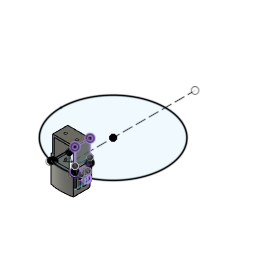
Aquazepp_Relais_Holder v4 (Autodesk Fusion 360 design; units mm, degrees)
Autodesk Fusion 360 part; units mm, degrees
sketch "Skizze1" plane through (0, 0, 0) normal (0, 0, 1) x (1, 0, 0)
  line L0 (-25.6418, 33.3344) -> (-25.6418, 4.3344)
  line L1 (-25.6418, 4.3344) -> (11.3582, 4.3344)
  line L2 (11.3582, 4.3344) -> (11.3582, 33.3344)
  line L3 (-28.6418, 33.3344) -> (-28.6418, 1.3344)
  line L4 (-28.6418, 1.3344) -> (14.3582, 1.3344)
  line L5 (14.3582, 1.3344) -> (14.3582, 33.3344)
  line L6 (-28.6418, 33.3344) -> (-25.6418, 33.3344)
  line L7 (11.3582, 33.3344) -> (14.3582, 33.3344)
  dimension "d1" = 29
  dimension "d2" = 37
  dimension "d3" = 29
  dimension "d4" = 3
  constraint vertical L0
  constraint perpendicular L0 L1
  constraint perpendicular L1 L2
  constraint perpendicular L0 L6
  measures "d1" distance of L0.start L0.end
  measures "d2" distance of L0.end L1.end
  measures "d3" distance of L1.end L2.end
extrude "Extrusion1" add sketch "Skizze1" along normal blind 39 makes body 1
sketch "Skizze2" plane through (14.3582, 0, 0) normal (1, 0, 0) x (0, 1, 0)
  line L0 (1.3344, 0) -> (33.3344, 0)
  line L1 (33.3344, 0) -> (33.3344, 39)
  line L2 (33.3344, 39) -> (1.3344, 39)
  line L3 (1.3344, 39) -> (1.3344, 0)
  line L4 (1.3344, 39) -> (33.3344, 39)
  line L5 (1.3344, 0) -> (1.3344, 39)
  line L6 (1.3344, 0) -> (33.3344, 0)
  line L7 (33.3344, 0) -> (33.3344, 39)
  circle A0 centre (14.3344, 30) radius 2.5
  circle A1 centre (26.3344, 30) radius 2.5
  circle A2 centre (14.3344, 18) radius 2.5
  circle A3 centre (26.3344, 18) radius 2.5
  dimension "d7" = 5
  dimension "d10" = 12
  dimension "d11" = -12
  dimension "d12" = 9
  dimension "d13" = 13
  measures "d7" diameter of A0
  measures "d12" distance of L4 A0.centre
  measures "d13" distance of L5 A0.centre
sketch "Skizze3" plane through (-28.6418, 0, 0) normal (-1, 0, 0) x (0, -1, 0)
  line L0 (-33.3344, 0) -> (-1.3344, 0)
  line L1 (-1.3344, 0) -> (-1.3344, 39)
  line L2 (-1.3344, 39) -> (-33.3344, 39)
  line L3 (-33.3344, 39) -> (-33.3344, 0)
  circle A0 centre (-26.3344, 30) radius 2.5
  circle A1 centre (-14.3344, 18) radius 2.5
extrude "Extrusion2" cut sketch "Skizze2" against normal blind 5 contours A0 | A3 bodies 1
extrude "Extrusion3" cut sketch "Skizze3" against normal blind 5 contours A0 | A1 bodies 1
sketch "Skizze4" plane through (0, 0, 39) normal (0, 0, 1) x (-1, 0, 0)
  line L0 (28.6418, -33.3344) -> (28.6418, -1.3344)
  line L1 (28.6418, -1.3344) -> (-14.3582, -1.3344)
  line L2 (-14.3582, -1.3344) -> (-14.3582, -33.3344)
  line L3 (-14.3582, -33.3344) -> (-11.3582, -33.3344)
  line L4 (-11.3582, -33.3344) -> (-11.3582, -4.3344)
  line L5 (-11.3582, -4.3344) -> (25.6418, -4.3344)
  line L6 (25.6418, -4.3344) -> (25.6418, -33.3344)
  line L7 (25.6418, -33.3344) -> (28.6418, -33.3344)
  circle A0 centre (7.1418, -99.3344) radius 100.5
  line L8 (25.6418, -33.3344) -> (-11.3582, -4.3344) construction
  line L9 (-11.3582, -33.3344) -> (25.6418, -4.3344) construction
  line L10 (7.1418, -18.8344) -> (7.1418, -257.1246) construction
  line L11 (28.6418, -1.3344) -> (28.6418, 1.2)
  line L12 (-14.3582, -1.3344) -> (-14.3582, 1)
  dimension "d18" = 201
  dimension "d19" = 98
  constraint coincident L6.end L7.start
  constraint coincident L4.end L5.start
  constraint coincident L3.end L4.start
  constraint coincident L5.end L6.start
  constraint midpoint L9 L10.start
  constraint perpendicular L5 L10
  constraint coincident A0.centre L10
  constraint coincident L0.end L1.start
  constraint perpendicular L1 L11
  constraint coincident L1.end L2.start
  constraint perpendicular L1 L12
  measures "d18" diameter of A0
  measures "d19" distance of L1 A0.centre
extrude "Extrusion4" add sketch "Skizze4" against normal blind 39 contours L1 A0 L11 L12 bodies 1
ref_plane "Arbeitsebene1" through (-7.1418, 12.8935, 41) normal (0, 0, 1) x (1, 0, 0)
sketch "Skizze5" plane through (-7.1418, 12.8935, 41) normal (0, 0, 1) x (1, 0, 0)
  line L0 (-18.5, 20.4409) -> (-18.5, -8.5591)
  line L1 (18.5, -8.5591) -> (18.5, 20.4409)
  line L2 (-21.5, 20.4409) -> (-21.5, -11.5591)
  line L3 (-21.5, -11.5591) -> (21.5, -11.5591)
  line L4 (-18.5, -8.5591) -> (18.5, -8.5591)
  line L5 (18.5, 20.4409) -> (21.5, 20.4409)
  line L6 (-21.5, 20.4409) -> (-18.5, 20.4409)
  line L7 (21.5, -11.5591) -> (21.5, 20.4409)
  line L8 (-18.5, -8.5591) -> (-21.5, -8.5591)
  line L9 (18.5, -8.5591) -> (21.5, -8.5591)
  constraint coincident L0.end L4.start
  constraint coincident L2 L8.end
  constraint perpendicular L2 L8
  constraint coincident L1.start L4.end
  constraint coincident L7 L9.end
  constraint perpendicular L7 L9
extrude "Extrusion5" add sketch "Skizze5" along normal blind 40 separate body contours L0 L2 L6 L8 | L1 L5 L7 L9 makes body 2 at (-25.6418, 14.001, 67.6667) makes body 3 at (11.3582, 23.6677, 67.6667)
sketch "Skizze6" plane through (0, 0, 81) normal (0, 0, 1) x (-1, 0, 0)
  line L0 (28.6418, -33.3344) -> (28.6418, -4.3344)
  line L1 (-14.3582, -4.3344) -> (-14.3582, -33.3344)
  line L2 (-14.3582, -33.3344) -> (-11.3582, -33.3344)
  line L3 (-11.3582, -33.3344) -> (-11.3582, -4.3344)
  line L4 (25.6418, -4.3344) -> (25.6418, -33.3344)
  line L5 (25.6418, -33.3344) -> (28.6418, -33.3344)
  line L6 (-14.3582, -1.3344) -> (-14.3582, -33.3344)
  line L7 (-11.3582, -4.3344) -> (-11.3582, -33.3344)
  line L8 (-11.3582, -33.3344) -> (-14.3582, -33.3344)
  line L9 (28.6418, -33.3344) -> (25.6418, -33.3344)
  line L10 (28.6418, -33.3344) -> (28.6418, -1.3344)
  line L11 (25.6418, -33.3344) -> (25.6418, -4.3344)
  line L12 (25.6418, -4.3344) -> (-11.3582, -4.3344)
  line L13 (28.6418, -1.3344) -> (-14.3582, -1.3344)
  line L14 (25.6418, -33.3344) -> (-11.3582, -33.3344)
  line L15 (-11.3582, -4.3344) -> (-14.3582, -4.3344)
  line L16 (28.6418, -4.3344) -> (25.6418, -4.3344)
  circle A0 centre (-3.6582, -18.7894) radius 2.5
  line L17 (25.6418, -33.3344) -> (-11.3582, -4.3344) construction
  line L18 (-11.3582, -33.3344) -> (25.6418, -4.3344) construction
  line L19 (7.1418, -18.8344) -> (7.1418, -24) construction
  line L20 (7.1418, -18.8344) -> (0, -18.8344) construction
  circle A1 centre (17.9418, -18.7894) radius 2.5
  dimension "d29" = 5
  dimension "d32" = 5
  dimension "d33" = 21.6
  constraint coincident L4.end L5.start
  constraint coincident L2.end L3.start
  constraint coincident L3.end L7.start
  constraint coincident L4.start L11.end
  constraint midpoint L18 L19.start
  constraint parallel L11 L19
  constraint perpendicular L19 L20
  constraint symmetric A0 L19 A1
  measures "d29" diameter of A0
  measures "d32" diameter of A1
  measures "d33" distance of A0.centre A1.centre
extrude "Extrusion6" add sketch "Skizze6" against normal blind 3 contours L3 L4 L7 L11 L12 L14 bodies 2 3
extrude "Extrusion7" add sketch "Skizze6" 1 faces at (-10.4374, 29.2618, 81) along normal blind 1 contours A0 | A1 on bodies 2 bodies 2
sketch "Skizze7" plane through (14.3582, 0, 0) normal (1, 0, 0) x (0, 1, 0)
  line L0 (4.3344, 41) -> (33.3344, 41)
  line L1 (33.3344, 41) -> (33.3344, 82)
  line L2 (33.3344, 82) -> (4.3344, 82)
  line L3 (4.3344, 82) -> (4.3344, 41)
  line L4 (4.3344, 41) -> (4.3344, 82)
  line L5 (33.3344, 41) -> (33.3344, 82)
  circle A0 centre (14.3344, 30) radius 2.5
  circle A1 centre (26.3344, 18) radius 2.5
  line L6 (4.3344, 41) -> (4.3344, 11)
  line L7 (33.3344, 41) -> (33.3344, 11)
  line L8 (33.3344, 11) -> (4.3344, 11)
  line L9 (11.8344, 30) -> (11.8344, 11)
  circle A2 centre (26.3344, 30) radius 2.5
  circle A3 centre (26.3344, 18) radius 2.5
  line L10 (16.8344, 30.0061) -> (16.8804, 11)
  line L11 (23.8344, 30.0061) -> (23.7883, 11)
  line L12 (28.8344, 30.0061) -> (28.8804, 11)
  line L13 (4.3344, 50.1435) -> (33.3344, 50.1435)
  constraint coincident L0.start L3.end
  constraint perpendicular L0 L6
  constraint coincident L0.end L1.start
  constraint parallel L4 L7
  constraint perpendicular L6 L8
  constraint coincident A0 L9.start
  constraint coincident L8 L9.end
  constraint tangent A0 L9
  constraint perpendicular L8 L9
  constraint coincident A0 L10.start
  constraint coincident L8 L10.end
  constraint tangent A0 L10
  constraint coincident A2 L11.start
  constraint coincident L8 L11.end
  constraint tangent A2 L11
  constraint coincident A2 L12.start
  constraint coincident L8 L12.end
  constraint tangent A2 L12
  constraint coincident L3 L13.start
  constraint coincident L1 L13.end
  constraint perpendicular L1 L13
extrude "Extrusion8" add sketch "Skizze7" along normal blind 3 separate body contours L0 L1 L3 L4 L5 L13 | L0 A0 L6 L7 L8 L9 A2 L10 L11 L12 makes body 4
sketch "Skizze8" plane through (-28.6418, 0, 0) normal (-1, 0, 0) x (0, -1, 0)
  line L0 (-33.3344, 41) -> (-4.3344, 41)
  line L1 (-4.3344, 41) -> (-4.3344, 82)
  line L2 (-4.3344, 82) -> (-33.3344, 82)
  line L3 (-33.3344, 82) -> (-33.3344, 41)
  line L4 (-4.3344, 50.1435) -> (-33.3344, 50.1435)
  line L5 (-33.3344, 41) -> (-33.3344, 82)
  line L6 (-4.3344, 41) -> (-4.3344, 82)
  line L7 (-4.3344, 41) -> (-4.3344, 11)
  line L8 (-33.3344, 41) -> (-33.3344, 11)
  circle A0 centre (-26.3344, 30) radius 2.5
  line L9 (-28.8344, 30.0061) -> (-28.8804, 11)
  line L10 (-23.8344, 30.0061) -> (-23.7883, 11)
  circle A1 centre (-14.3344, 30) radius 2.5
  line L11 (-16.8344, 30.0061) -> (-16.8804, 11)
  line L12 (-11.8344, 30) -> (-11.8344, 11)
  line L13 (-33.3344, 11) -> (-4.3344, 11)
extrude "Extrusion9" add sketch "Skizze8" along normal blind 3 separate body contours L0 L1 L3 L4 L5 L6 | L0 L7 L8 A0 L9 L10 A1 L11 L12 L13 makes body 5
combine "Kombinieren1" operation add target body 2 tool bodies 5 4
fillet "Abrundung1" radius 4 12 edges at (12.8582, 33.3344, 39) (12.8582, 33.3344, 0) (-27.1418, 33.3344, 0) (-27.1418, 33.3344, 39) (-27.1418, 4.3344, 41) (12.8582, 4.3344, 41) (12.8582, 33.3344, 41) (-27.1418, 33.3344, 41) (15.8582, 4.3344, 11) (15.8582, 33.3344, 11) (-30.1418, 33.3344, 11) (-30.1418, 4.3344, 11) on bodies 1 2
fillet "Abrundung1" radius 3 2 edges at (-31.6418, 18.8344, 50.1435) (17.3582, 18.8344, 50.1435) on bodies 1 2
fillet "Abrundung1" radius 2 2 edges at (-25.6418, 18.8344, 41) (11.3582, 18.8344, 41) on bodies 1 2
equation "d3 = d1"
named bodies: "RelaisHolder", "RelaisCap"
